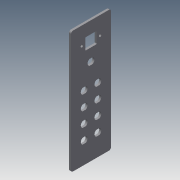
# Autodesk Inventor part: Front-panel
Saved by Autodesk Inventor 2015 SP1 (Build 190203100, 203)
## iProperties
Created: 2015-07-22
Part Number: Front-panel
Material: Generic
Document SubType Name: Modeling
Designer: James
Density: 1 g/cm^3
Appearance: Default
Author: James
Autodesk Inventor part; units mm, degrees
ref_plane "YZ Plane" through (0, 0, 0) normal (1, 0, 0) x (0, 1, 0)
ref_plane "XZ Plane" through (0, 0, 0) normal (0, 1, 0) x (-1, 0, 0)
ref_plane "XY Plane" through (0, 0, 0) normal (0, 0, 1) x (1, 0, 0)
sketch "Sketch1" plane through (0, 0, 0) normal (1, 0, 0) x (0, 1, 0)
  line L0 (29.6568, 89.9307) -> (-25.9432, 89.9307)
  line L1 (-25.9432, 89.9307) -> (-25.9432, -79.5693)
  line L2 (-25.9432, -79.5693) -> (29.6568, -79.5693)
  line L3 (29.6568, -79.5693) -> (29.6568, 89.9307)
  point P0 (0, 0)
  dimension "d0" = 169.5
  dimension "d1" = 55.6
  constraints: 8 end point, 2 parallel, 1 horizontal, 1 perpendicular
  measures "d0" distance between parallel lines of L0 L2
  measures "d1" distance between parallel lines of L3 L1
extrude "Extrusion1" add sketch "Sketch1" along normal blind 3
fillet "Fillet1" radius 3 4 edges at (1.5, 29.6568, 89.9307) (1.5, -25.9432, 89.9307) (1.5, 29.6568, -79.5693) (1.5, -25.9432, -79.5693)
sketch "Sketch2" plane through (3, 0, 0) normal (1, 0, 0) x (0, 0, -1)
  line L0 (-80.1807, 24.3568) -> (69.8193, 24.3568)
  line L1 (69.8193, 24.3568) -> (69.8193, -20.6432)
  line L2 (69.8193, -20.6432) -> (-80.1807, -20.6432)
  line L3 (-80.1807, -20.6432) -> (-80.1807, 24.3568)
  line L4 (-89.9307, 26.6568) -> (-89.9307, -22.9432) projected
  line L5 (79.5693, -22.9432) -> (79.5693, 26.6568) projected
  line L6 (-86.9307, -25.9432) -> (76.5693, -25.9432) projected
  line L7 (76.5693, 29.6568) -> (-86.9307, 29.6568) projected
  point P0 (0, 0)
  dimension "d5" = 150
  dimension "d6" = 45
  dimension "d9" = 169.5
  dimension "d10" = 9.75
  dimension "d11" = 55.6
  dimension "d12" = 5.3
  constraints: 8 end point, 2 parallel, 1 horizontal, 1 perpendicular
  measures "d5" distance between parallel lines of L3 L1
  measures "d6" distance between parallel lines of L2 L0
  measures "d9" distance between parallel lines of L4 L5
  measures "d10" distance between parallel lines of L5 L1
  measures "d11" distance between parallel lines of L6 L7
  measures "d12" distance between parallel lines of L7 L0
extrude "Extrusion2" cut sketch "Sketch2" against normal blind 0.1
sketch "Sketch4" plane through (2.9, 0, 0) normal (1, 0, 0) x (0, 0, -1)
  line L0 (-80.1807, 24.3568) -> (69.8193, 24.3568)
  line L1 (69.8193, 24.3568) -> (69.8193, -20.6432)
  line L2 (69.8193, -20.6432) -> (-80.1807, -20.6432)
  line L3 (-80.1807, -20.6432) -> (-80.1807, 24.3568)
  line L4 (-44.3307, 4.1676) -> (-36.0307, 4.1676)
  line L5 (-36.0307, 4.1676) -> (-36.0307, -0.4541)
  line L6 (-36.0307, -0.4541) -> (-44.3307, -0.4541)
  line L7 (-44.3307, -0.4541) -> (-44.3307, 4.1676)
  line L8 (-44.3307, 4.1676) -> (-36.0307, -0.4541) construction
  line L9 (-36.0307, 4.1676) -> (-44.3307, -0.4541) construction
  arc A0 (-36.0307, 4.1676) -> (-44.3307, 4.1676) centre (-40.1807, 1.8568) ccw
  line L10 (-14.3307, 9.0459) -> (-6.0307, 9.0459)
  line L11 (-6.0307, 9.0459) -> (-6.0307, 13.6676)
  line L12 (-6.0307, 13.6676) -> (-14.3307, 13.6676)
  line L13 (-14.3307, 13.6676) -> (-14.3307, 9.0459)
  line L14 (-14.3307, 9.0459) -> (-6.0307, 13.6676) construction
  line L15 (-6.0307, 9.0459) -> (-14.3307, 13.6676) construction
  arc A1 (-6.0307, 13.6676) -> (-14.3307, 13.6676) centre (-10.1807, 11.3568) ccw
  arc A2 (-14.3307, 9.0459) -> (-6.0307, 9.0459) centre (-10.1807, 11.3568) ccw
  line L16 (5.6693, 13.6676) -> (13.9693, 13.6676)
  line L17 (13.9693, 13.6676) -> (13.9693, 9.0459)
  line L18 (13.9693, 9.0459) -> (5.6693, 9.0459)
  line L19 (5.6693, 9.0459) -> (5.6693, 13.6676)
  line L20 (5.6693, 13.6676) -> (13.9693, 9.0459) construction
  line L21 (13.9693, 13.6676) -> (5.6693, 9.0459) construction
  arc A3 (13.9693, 13.6676) -> (5.6693, 13.6676) centre (9.8193, 11.3568) ccw
  arc A4 (5.6693, 9.0459) -> (13.9693, 9.0459) centre (9.8193, 11.3568) ccw
  line L22 (25.6693, 9.0459) -> (33.9693, 9.0459)
  line L23 (33.9693, 9.0459) -> (33.9693, 13.6676)
  line L24 (33.9693, 13.6676) -> (25.6693, 13.6676)
  line L25 (25.6693, 13.6676) -> (25.6693, 9.0459)
  line L26 (25.6693, 9.0459) -> (33.9693, 13.6676) construction
  line L27 (33.9693, 9.0459) -> (25.6693, 13.6676) construction
  line L28 (53.9693, -9.9541) -> (45.6693, -9.9541)
  line L29 (45.6693, -9.9541) -> (45.6693, -5.3324)
  line L30 (45.6693, -5.3324) -> (53.9693, -5.3324)
  line L31 (53.9693, -5.3324) -> (53.9693, -9.9541)
  line L32 (53.9693, -9.9541) -> (45.6693, -5.3324) construction
  line L33 (45.6693, -9.9541) -> (53.9693, -5.3324) construction
  line L34 (25.6693, -9.9541) -> (33.9693, -9.9541)
  line L35 (33.9693, -9.9541) -> (33.9693, -5.3324)
  line L36 (33.9693, -5.3324) -> (25.6693, -5.3324)
  line L37 (25.6693, -5.3324) -> (25.6693, -9.9541)
  line L38 (25.6693, -9.9541) -> (33.9693, -5.3324) construction
  line L39 (33.9693, -9.9541) -> (25.6693, -5.3324) construction
  line L40 (13.9693, -9.9541) -> (5.6693, -9.9541)
  line L41 (5.6693, -9.9541) -> (5.6693, -5.3324)
  line L42 (5.6693, -5.3324) -> (13.9693, -5.3324)
  line L43 (13.9693, -5.3324) -> (13.9693, -9.9541)
  line L44 (13.9693, -9.9541) -> (5.6693, -5.3324) construction
  line L45 (5.6693, -9.9541) -> (13.9693, -5.3324) construction
  line L46 (-14.3307, -9.9541) -> (-6.0307, -9.9541)
  line L47 (-6.0307, -9.9541) -> (-6.0307, -5.3324)
  line L48 (-6.0307, -5.3324) -> (-14.3307, -5.3324)
  line L49 (-14.3307, -5.3324) -> (-14.3307, -9.9541)
  line L50 (-14.3307, -9.9541) -> (-6.0307, -5.3324) construction
  line L51 (-6.0307, -9.9541) -> (-14.3307, -5.3324) construction
  arc A5 (-6.0307, -5.3324) -> (-14.3307, -5.3324) centre (-10.1807, -7.6432) ccw
  arc A6 (-14.3307, -9.9541) -> (-6.0307, -9.9541) centre (-10.1807, -7.6432) ccw
  arc A7 (13.9693, -5.3324) -> (5.6693, -5.3324) centre (9.8193, -7.6432) ccw
  arc A8 (5.6693, -9.9541) -> (13.9693, -9.9541) centre (9.8193, -7.6432) ccw
  arc A9 (33.9693, -5.3324) -> (25.6693, -5.3324) centre (29.8193, -7.6432) ccw
  arc A10 (25.6693, -9.9541) -> (33.9693, -9.9541) centre (29.8193, -7.6432) ccw
  arc A11 (53.9693, -5.3324) -> (45.6693, -5.3324) centre (49.8193, -7.6432) ccw
  arc A12 (45.6693, -9.9541) -> (53.9693, -9.9541) centre (49.8193, -7.6432) ccw
  arc A13 (33.9693, 13.6676) -> (25.6693, 13.6676) centre (29.8193, 11.3568) ccw
  arc A14 (25.6693, 9.0459) -> (33.9693, 9.0459) centre (29.8193, 11.3568) ccw
  line L52 (53.9693, 9.0459) -> (45.6693, 9.0459)
  line L53 (45.6693, 9.0459) -> (45.6693, 13.6676)
  line L54 (45.6693, 13.6676) -> (53.9693, 13.6676)
  line L55 (53.9693, 13.6676) -> (53.9693, 9.0459)
  line L56 (53.9693, 9.0459) -> (45.6693, 13.6676) construction
  line L57 (45.6693, 9.0459) -> (53.9693, 13.6676) construction
  arc A15 (53.9693, 13.6676) -> (45.6693, 13.6676) centre (49.8193, 11.3568) ccw
  arc A16 (45.6693, 9.0459) -> (53.9693, 9.0459) centre (49.8193, 11.3568) ccw
  arc A17 (-44.3307, -0.4541) -> (-36.0307, -0.4541) centre (-40.1807, 1.8568) ccw
  line L58 (-73.1807, -6.1432) -> (-73.1807, 9.8568)
  line L59 (-73.1807, 9.8568) -> (-57.1807, 9.8568)
  line L60 (-57.1807, 9.8568) -> (-57.1807, -6.1432)
  line L61 (-57.1807, -6.1432) -> (-73.1807, -6.1432)
  line L62 (-73.1807, -6.1432) -> (-57.1807, 9.8568) construction
  line L63 (-73.1807, 9.8568) -> (-57.1807, -6.1432) construction
  point P0 (0, 0)
  point P1 (-65.1807, 1.8568)
  point P2 (-65.1807, -10.8432)
  point P3 (-65.1807, 14.5568)
  dimension "d16" = 20
  dimension "d17" = 20
  dimension "d18" = 20
  dimension "d20" = 19
  dimension "d25" = 20
  dimension "d26" = 20
  dimension "d27" = 20
  dimension "d28" = 19
  dimension "d29" = 19
  dimension "d43" = 13
  dimension "d44" = 45
  dimension "d45" = 13
  dimension "d46" = 13
  dimension "d47" = 13
  dimension "d70" = 22.5
  dimension "d71" = 8.3
  dimension "d72" = 4.75
  dimension "d73" = 40
  dimension "d74" = 20.1892
  dimension "d75" = 8.3
  dimension "d76" = 4.75
  dimension "d77" = 8.3
  dimension "d78" = 4.75
  dimension "d79" = 8.3
  dimension "d81" = 8.3
  dimension "d82" = 8.3
  dimension "d83" = 8.3
  dimension "d84" = 8.3
  dimension "d85" = 4.75
  dimension "d86" = 4.75
  dimension "d88" = 4.75
  dimension "d90" = 4.75
  dimension "d98" = 20
  dimension "d100" = 20
  dimension "d101" = 8.3
  dimension "d104" = 16
  dimension "d105" = 16
  dimension "d106" = 15
  dimension "d107" = 22.5
  dimension "d108" = 8
  dimension "d109" = 8
  dimension "d110" = 12.7
  dimension "d111" = 12.7
  constraints: 128 end point, 36 point on circle, 24 midpoint, 22 parallel, 18 centre point, 15 coincident, 11 perpendicular, 10 horizontal, 1 vertical
  measures "d16" distance of point (49.819, 11.357) point (29.819, 11.357)
  measures "d17" distance of point (9.819, 11.357) point (29.819, 11.357)
  measures "d18" distance of point (9.819, 11.357) point (-10.181, 11.357)
  measures "d20" distance of point (-10.181, 11.357) point (-10.181, -7.643)
  measures "d25" distance of point (49.819, -7.643) point (29.819, -7.643)
  measures "d26" distance of point (9.819, -7.643) point (29.819, -7.643)
  measures "d27" distance of point (-10.181, -7.643) point (9.819, -7.643)
  measures "d28" distance of point (9.819, -7.643) point (9.819, 11.357)
  measures "d29" distance of point (29.819, 11.357) point (29.819, -7.643)
  measures "d43" distance from line of point (-10.181, -7.643) L2
  measures "d44" distance of L2.end L0.start
  measures "d45" distance from line of L2 point (9.819, -7.643)
  measures "d46" distance from line of L2 point (29.819, -7.643)
  measures "d47" distance from line of L2 point (49.819, -7.643)
  measures "d70" distance from line of point (-40.181, 1.857) L0
  measures "d71" distance between parallel lines of L5 L7
  measures "d72" radius of A0
  measures "d73" distance from line of A0.centre L3
  measures "d74" distance between parallel lines of L0 L4
  measures "d75" distance between parallel lines of L11 L13
  measures "d76" radius of A2
  measures "d77" distance between parallel lines of L19 L17
  measures "d78" radius of A3
  measures "d79" distance between parallel lines of L25 L23
  measures "d81" distance between parallel lines of L31 L29
  measures "d82" distance between parallel lines of L37 L35
  measures "d83" distance between parallel lines of L43 L41
  measures "d84" distance between parallel lines of L47 L49
  measures "d85" radius of A6
  measures "d86" radius of A7
  measures "d88" radius of A10
  measures "d90" radius of A13
  measures "d98" distance from line of L1 A11.centre
  measures "d100" distance from line of L1 point (49.819, 11.357)
  measures "d101" distance between parallel lines of L55 L53
  measures "d104" distance between parallel lines of L60 L58
  measures "d105" distance between parallel lines of L61 L59
  measures "d106" distance from line of point (-65.181, 1.857) L3
  measures "d107" distance from line of point (-65.181, 1.857) L2
  measures "d108" distance from line of point (-65.181, 14.557) L60
  measures "d109" distance from line of L60 point (-65.181, -10.843)
  measures "d110" distance of point (-65.181, 1.857) point (-65.181, -10.843)
  measures "d111" distance of point (-65.181, 14.557) point (-65.181, 1.857)
extrude "Extrusion3" cut sketch "Sketch4" against normal blind 20 contours A0 L4 | L4 L5 L6 L7 | L6 A17 | L13 L12 L11 L10 | L10 A2 | A1 L12 | A3 L16 | L16 L17 L18 L19 | L18 A4 | L25 L24 L23 L22 | L22 A14 | A13 L24 | A12 L28 | L28 L29 L30 L31 | L30 A11 | L37 L36 L35 L34 | L34 A10 | A9 L36 | A8 L40 | L40 L41 L42 L43 | L42 A7 | L49 L48 L47 L46 | L46 A6 | A5 L48 | A16 L52 | L52 L53 L54 L55 | L54 A15 | L58 L59 L60 L61
fillet "Fillet2" radius 1 4 edges at (1.45, 9.8568, 57.1807) (1.45, -6.1432, 57.1807) (1.45, -6.1432, 73.1807) (1.45, 9.8568, 73.1807)
hole "Hole4" at (2.9, 1.8568, 40.1807) at (2.9, 11.3568, -9.8193) at (2.9, 11.3568, 10.1807) at (2.9, 11.3568, -29.8193) at (2.9, 11.3568, -49.8193) at (2.9, -7.6432, 10.1807) at (2.9, -7.6432, -9.8193) at (2.9, -7.6432, -29.8193) at (2.9, -7.6432, -49.8193) at (2.9, -10.8432, 65.1807) at (2.9, 14.5568, 65.1807) direction (-1, 0, 0) diameter 3.4 end through all clearance for "Flat Head Machine Screw" size "M3" standard "Ansi Metric M Profile"
sketch "Sketch9" plane through (3, 0, 0) normal (1, 0, 0) x (0, 0, -1)
  line L0 (-80.1807, -20.6432) -> (-80.1807, 24.3568) projected
  line L1 (-80.1807, 24.3568) -> (69.8193, 24.3568) projected
  line L2 (69.8193, 24.3568) -> (69.8193, -20.6432) projected
  line L3 (69.8193, -20.6432) -> (-80.1807, -20.6432) projected
  arc A0 (76.5693, -25.9432) -> (79.5693, -22.9432) centre (76.5693, -22.9432) ccw projected
  line L4 (79.5693, -22.9432) -> (79.5693, 26.6568) projected
  arc A1 (79.5693, 26.6568) -> (76.5693, 29.6568) centre (76.5693, 26.6568) ccw projected
  line L5 (76.5693, 29.6568) -> (-86.9307, 29.6568) projected
  arc A2 (-86.9307, 29.6568) -> (-89.9307, 26.6568) centre (-86.9307, 26.6568) ccw projected
  line L6 (-89.9307, 26.6568) -> (-89.9307, -22.9432) projected
  arc A3 (-89.9307, -22.9432) -> (-86.9307, -25.9432) centre (-86.9307, -22.9432) ccw projected
  line L7 (-86.9307, -25.9432) -> (76.5693, -25.9432) projected
  point P0 (0, 0)
extrude "Extrusion4" cut sketch "Sketch9" against normal blind 0.1
equation "\"d10\" = -0.5 * d5 + 0.5 * d9"
equation "\"d12\" = -0.5 * d6 + 0.5 * d11"
equation "\"d25\" = d16"
equation "\"d26\" = d17"
equation "\"d27\" = d18"
equation "\"d28\" = d20"
equation "\"d29\" = d28"
equation "\"d43\" = -0.5 * d20 + 0.5 * d44"
equation "\"d45\" = d43"
equation "\"d46\" = d45"
equation "\"d47\" = d46"
equation "\"d78\" = d76"
equation "\"d85\" = d76"
equation "\"d86\" = d85"
equation "\"d88\" = d86"
equation "\"d90\" = d78"
body "Solid1"
